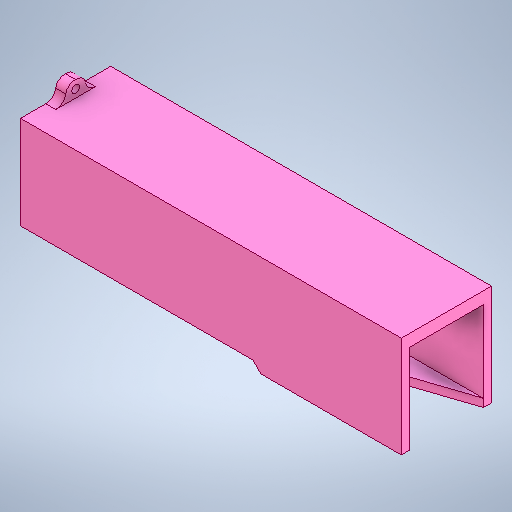
# Autodesk Inventor part: PipetteStand
Saved by Autodesk Inventor 2025.1 (Build 291241000, 241)
## iProperties
Created: 2024-11-06
Part Number: PipetteStand
Material: Generic
Document SubType Name: Modeling
Designer: 13156
Density: 1 g/cm^3
Appearance: Default
Author: 13156
Autodesk Inventor part; units mm, degrees
ref_plane "YZ Plane" through (0, 0, 0) normal (1, 0, 0) x (0, 1, 0)
ref_plane "XZ Plane" through (0, 0, 0) normal (0, 1, 0) x (-1, 0, 0)
ref_plane "XY Plane" through (0, 0, 0) normal (0, 0, 1) x (1, 0, 0)
sketch "Sketch2" plane through (0, 0, 0) normal (1, 0, 0) x (0, 1, 0)
  line L0 (26, 22.5) -> (-26, 22.5)
  line L1 (-26, 22.5) -> (-26, -22.5)
  line L2 (-26, -22.5) -> (26, -22.5)
  line L3 (26, -22.5) -> (26, 22.5)
  point P0 (0, 0)
  point P1 (-26, 0)
  point P2 (26, 0)
  dimension "d0" = 45
  dimension "d1" = 52
  dimension "d2" = 26
  dimension "d3" = 22.5
  constraints: 8 end point, 2 midpoint, 2 parallel, 1 horizontal, 1 perpendicular
  measures "d0" distance between parallel lines of L2 L0
  measures "d1" distance from line of point (-26, 0) L3
  measures "d2" distance of point (0, 0) point (26, 0)
  measures "d3" distance from line of point (0, 0) L2
extrude "Extrusion1" add sketch "Sketch2" along normal blind 125.1
sketch "Sketch3" plane through (0, -26, -22.5) normal (0, -1, 0) x (1, 0, 0)
  line L0 (125.1, 45) -> (125.1, 0) projected
  line L1 (125.1, 41) -> (5, 41)
  line L2 (5, 41) -> (5, 4)
  line L3 (5, 4) -> (125.1, 4)
  line L4 (125.1, 4) -> (125.1, 41)
  line L5 (0, 45) -> (0, 0) projected
  line L6 (0, 0) -> (125.1, 0) projected
  line L7 (0, 45) -> (125.1, 45) projected
  point P0 (0, 22.5)
  point P1 (125.1, 4)
  dimension "d6" = 5
  dimension "d7" = 37
  dimension "d8" = 4
  dimension "d45" = 4
  constraints: 8 end point, 2 parallel, 1 horizontal, 1 perpendicular, 1 point on line
  measures "d6" distance between parallel lines of L5 L2
  measures "d7" distance between parallel lines of L3 L1
  measures "d8" distance between parallel lines of L6 L3
  measures "d45" distance between parallel lines of L7 L1
extrude "Extrusion2" cut sketch "Sketch3" against normal blind 40.5 contours L0 L3 L2 L1
sketch "Sketch4" plane through (0, 0, 0) normal (-1, 0, 0) x (0, 0, 1)
  line L0 (22.5, -26) -> (18.5, -26) projected
  line L1 (-22.5, 26) -> (22.5, 26) projected
  line L2 (22.5, -26) -> (-22.5, -26)
  line L3 (-22.5, -26) -> (-22.5, 26)
  line L4 (-22.5, 26) -> (22.5, 26)
  line L5 (22.5, 26) -> (22.5, -26)
  line L6 (17.5, -26) -> (-17.5, -26)
  line L7 (-17.5, -26) -> (-17.5, 21)
  line L8 (-17.5, 21) -> (17.5, 21)
  line L9 (17.5, 21) -> (17.5, -26)
  point P0 (0, 0)
  point P1 (-17.5, -26)
  point P2 (22.5, 26)
  dimension "d11" = 5
  dimension "d12" = 5
  dimension "d13" = 5
  constraints: 16 end point, 4 parallel, 2 horizontal, 2 perpendicular, 1 point on line
  measures "d11" distance between parallel lines of L5 L9
  measures "d12" distance between parallel lines of L3 L7
  measures "d13" distance between parallel lines of L1 L8
extrude "Extrusion3" add sketch "Sketch4" along normal blind 120
sketch "Sketch5" plane through (0, 0, 0) normal (-1, 0, 0) x (0, 0, 1)
  line L0 (17.5, -26) -> (-17.5, -26) projected
  line L1 (11, -26) -> (-11, -26)
  line L2 (-11, -26) -> (-11, 9.5)
  line L3 (-11, 9.5) -> (11, 9.5)
  line L4 (11, 9.5) -> (11, -26)
  line L5 (17.5, 21) -> (17.5, -26) projected
  line L6 (-17.5, -26) -> (-17.5, 21) projected
  line L7 (-17.5, 21) -> (17.5, 21) projected
  point P0 (0, 0)
  point P1 (-11, -26)
  dimension "d16" = 6.5
  dimension "d17" = 6.5
  dimension "d18" = 11.5
  constraints: 8 end point, 2 parallel, 1 horizontal, 1 perpendicular, 1 point on line
  measures "d16" distance between parallel lines of L5 L4
  measures "d17" distance between parallel lines of L6 L2
  measures "d18" distance between parallel lines of L7 L3
extrude "Extrusion4" cut sketch "Sketch5" against normal blind 5 contours L0 L2 L3 L4
sketch "Sketch7" plane through (125.1, 0, 0) normal (1, 0, 0) x (0, 0, -1)
  line L0 (22.5, 26) -> (-22.5, 26) projected
  line L1 (22.5, -26) -> (22.5, 26) projected
  line L2 (-22.5, 26) -> (22.5, 26)
  line L3 (22.5, 26) -> (22.5, -26)
  line L4 (22.5, -26) -> (-22.5, -26)
  line L5 (-22.5, -26) -> (-22.5, 26)
  point P0 (0, 0)
  constraints: 8 end point, 2 parallel, 1 horizontal, 1 perpendicular
extrude "Extrusion6" cut sketch "Sketch7" against normal blind 55
sketch "Sketch12" plane through (0, 0, 0) normal (1, 0, 0) x (0, 0, -1)
  line L0 (-18.5, 14.5) -> (18.5, 14.5)
  line L1 (18.5, 14.5) -> (18.5, -26)
  line L2 (18.5, -26) -> (-18.5, -26)
  line L3 (-18.5, -26) -> (-18.5, 14.5)
  point P0 (0, 0)
  constraints: 8 end point, 2 parallel, 1 horizontal, 1 perpendicular
extrude "Extrusion11" cut sketch "Sketch12" against normal blind 115
sketch "Sketch13" plane through (-115, 0, 0) normal (1, 0, 0) x (0, 0, -1)
  circle A0 centre (0, 6.5) radius 1.95
  circle A1 centre (0, -18) radius 1.95
  line L0 (-18.5, 14.5) -> (18.5, 14.5) projected
  line L1 (18.5, -26) -> (-18.5, -26) projected
  point P0 (0, 0)
  dimension "d49" = 3.9
  dimension "d50" = 8
  dimension "d51" = 18.5
  dimension "d52" = 8
  dimension "d53" = 24.5
  constraints: 2 centre point, 1 equal radius
  measures "d49" diameter of A0
  measures "d50" distance from line of L0 A0.centre
  measures "d51" horizontal distance of L1.start A1.centre
  measures "d52" distance from line of L1 A1.centre
  measures "d53" distance of A1.centre A0.centre
extrude "Extrusion12" cut sketch "Sketch13" against normal blind 5
sketch "Sketch14" plane through (-120, -26, -22.5) normal (0, -1, 0) x (1, 0, 0)
  line L0 (190.1, 45) -> (0, 45) projected
  line L1 (190.1, 45) -> (120, 45)
  line L2 (0, 0) -> (190.1, 0) projected
  line L3 (120, 0) -> (120, 45)
  line L4 (120, 0) -> (190.1, 0)
  line L5 (190.1, 0) -> (190.1, 4.0746)
  line L6 (190.1, 4.0746) -> (190.1, 0)
  line L7 (190.1, 45) -> (190.1, 41)
  line L8 (190.1, 41) -> (150.1436, 27.692)
  line L9 (150.1436, 27.692) -> (150.1436, 17.308)
  line L10 (190.1, 4) -> (125, 4) projected
  line L11 (150.1436, 17.308) -> (190.1, 4)
  line L12 (120, 22.5) -> (198.6661, 22.5) construction
  line L13 (125, 4) -> (125, 11.5) projected
  point P0 (125, 7.75)
  dimension "d56" = 39.9564
  dimension "d57" = 5
  dimension "d58" = 13.308
  constraints: 20 end point, 3 point on line, 2 collinear, 2 perpendicular, 1 horizontal, 1 midpoint, 1 parallel, 1 other
  measures "d56" horizontal distance of L9.end L10.start
  measures "d57" distance from line of point (125, 7.75) L3
  measures "d58" vertical distance of L7.end L8.end
extrude "Extrusion13" add sketch "Sketch14" along normal blind 4
chamfer "Chamfer1" distance 4 angle 45 2 edges at (0, -26, 20.5) (0, -26, -20.5)
sketch "Sketch15" plane through (5, 14.5, 18.5) normal (1, 0, 0) x (0, 0, -1)
  line L0 (0, -40.5) -> (0, 0) projected
  line L1 (41, -40.5) -> (-4, -40.5) projected
  line L2 (0, -36) -> (36.9968, -36)
  line L3 (36.9968, -36) -> (36.9968, -40.5)
  line L4 (36.9968, -40.5) -> (0, -40.5)
  line L5 (0, -40.5) -> (0, -36)
  line L6 (7.5, -5) -> (29.5, -5) projected
  point P0 (18.5, -14.5)
  dimension "d64" = 31
  constraints: 8 end point, 2 parallel, 2 point on line, 1 horizontal, 1 perpendicular
  measures "d64" distance between parallel lines of L2 L6
extrude "Extrusion14" add sketch "Sketch15" against normal up to surface (5 mm away)
sketch "Sketch16" plane through (70.1, 0, 0) normal (1, 0, 0) x (0, 0, -1)
  line L0 (-22.5, -26) -> (-22.5, 26) projected
  line L1 (22.5, 26) -> (22.5, -26) projected
  line L2 (-22.5, 26) -> (22.5, 26)
  line L3 (22.5, 26) -> (22.5, 20.5)
  line L4 (22.5, 20.5) -> (-22.5, 20.5)
  line L5 (-22.5, 20.5) -> (-22.5, 26)
  line L6 (18.5, 14.5) -> (-18.5, 14.5) projected
  point P0 (0, 0)
  dimension "d67" = 6
  constraints: 8 end point, 2 parallel, 1 horizontal, 1 perpendicular, 1 point on line
  measures "d67" distance between parallel lines of L4 L6
extrude "Extrusion15" cut sketch "Sketch16" against normal blind 270.35
sketch "Sketch17" plane through (-120, 0, 0) normal (-1, 0, 0) x (0, 0, 1)
  line L0 (22.5, 20.5) -> (-22.5, 20.5) projected
  line L1 (-5, 20.5) -> (5, 20.5)
  line L2 (5, 20.5) -> (5, 28.5)
  line L3 (5, 28.5) -> (-5, 28.5)
  line L4 (-5, 28.5) -> (-5, 20.5)
  line L5 (18.5, -30) -> (-18.5, -30) construction
  line L6 (0, -30) -> (0, 42.9125) construction
  point P0 (0, 0)
  dimension "d70" = 10
  dimension "d71" = 8
  constraints: 10 end point, 2 parallel, 1 horizontal, 1 midpoint, 1 perpendicular, 1 point on line, 1 vertical, 1 other
  measures "d70" distance between parallel lines of L2 L4
  measures "d71" distance between parallel lines of L0 L3
extrude "Extrusion16" add sketch "Sketch17" against normal blind 5
sketch "Sketch18" plane through (-115, 0, 0) normal (1, 0, 0) x (0, 0, -1)
  circle A0 centre (0, 24.5) radius 1.95
  line L0 (22.5, 20.5) -> (-22.5, 20.5) projected
  line L1 (0, 20.5) -> (0, 34.3113)
  line L2 (-5, 28.5) -> (-5, 20.5) projected
  point P0 (0, 0)
  dimension "d74" = 3.9
  dimension "d75" = 4
  dimension "d76" = 5
  constraints: 2 end point, 1 centre point, 1 midpoint, 1 vertical
  measures "d74" diameter of A0
  measures "d75" distance from line of L0 A0.centre
  measures "d76" distance from line of L2 A0.centre
extrude "Extrusion17" cut sketch "Sketch18" against normal blind 5
fillet "Fillet2" radius 5 2 edges at (-117.5, 28.5, -5) (-117.5, 28.5, 5) curvature continuous yes
fillet "Fillet3" radius 5 2 edges at (-117.5, 20.5, 5) (-117.5, 20.5, -5)
sketch "Sketch19" plane through (-120, 0, 0) normal (-1, 0, 0) x (0, 0, 1)
  line L0 (-22.5, -26) -> (22.5, -26) projected
  line L1 (5, -26) -> (-5, -26)
  line L2 (-5, -26) -> (-5, -34)
  line L3 (-5, -34) -> (5, -34)
  line L4 (5, -34) -> (5, -26)
  circle A0 centre (0, -30) radius 1.95
  point P0 (0, 0)
  dimension "d81" = 10
  dimension "d82" = 8
  dimension "d83" = 5
  dimension "d84" = 3.9
  dimension "d85" = 4
  dimension "d86" = 30
  constraints: 8 end point, 2 parallel, 1 centre point, 1 horizontal, 1 perpendicular, 1 point on line
  measures "d81" distance between parallel lines of L2 L4
  measures "d82" distance of L1.end L2.end
  measures "d83" distance from line of point (0, 0) L4
  measures "d84" diameter of A0
  measures "d85" distance from line of L0 A0.centre
  measures "d86" distance of point (0, 0) A0.centre
extrude "Extrusion18" add sketch "Sketch19" against normal blind 5
fillet "Fillet4" radius 5 2 edges at (-117.5, -34, 5) (-117.5, -34, -5)
fillet "Fillet5" radius 5 2 edges at (-117.5, -26, -5) (-117.5, -26, 5)
body "Solid1"
